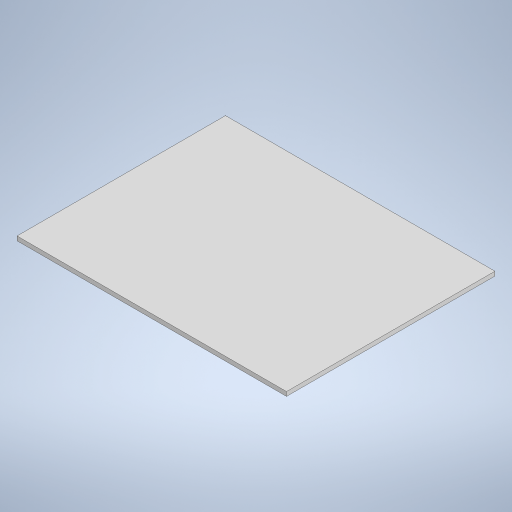
# Autodesk Inventor part: Sliding_Door
Saved by Autodesk Inventor 2024 (Build 280153000, 153)
## iProperties
Created: 2023-10-02
Part Number: Sliding_Door
Material: Generic
Document SubType Name: Modeling
Designer: vegaj
Density: 1 g/cm^3
Appearance: Default
Author: vegaj
Autodesk Inventor part; units mm, degrees
ref_plane "YZ Plane" through (0, 0, 0) normal (1, 0, 0) x (0, 1, 0)
ref_plane "XZ Plane" through (0, 0, 0) normal (0, 1, 0) x (-1, 0, 0)
ref_plane "XY Plane" through (0, 0, 0) normal (0, 0, 1) x (1, 0, 0)
sketch "Sketch1" plane through (0, 0, 0) normal (0, 1, 0) x (-1, 0, 0)
  line L0 (0, 0) -> (196.215, 0)
  line L1 (196.215, 0) -> (196.215, -151.765)
  line L2 (196.215, -151.765) -> (0, -151.765)
  line L3 (0, -151.765) -> (0, 0)
  dimension "d0" = 196.215
  dimension "d1" = 151.765
  constraints: 8 end point, 2 parallel, 1 horizontal, 1 perpendicular
  measures "d0" distance of L1.end L2.end
  measures "d1" distance of L0.end L1.end
extrude "Extrusion1" add sketch "Sketch1" along normal blind 3.048
body "Solid1"
